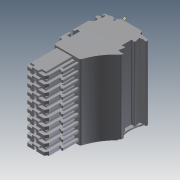
# Autodesk Inventor part: 2010-1201
Saved by Autodesk Inventor 2016 (Build 200138000, 138)
## iProperties
Created: 2014-05-05
Part Number: 2010-1201
Catalog Web Link: www.cadenas.de
Description: 2020-102 TO 2020-115-1-CONDUCTOR FEMALE PLUG for insertion into carrier terminal blocks WITH CODIG FINGERS
Vendor: WAGO
Document SubType Name: Modeling
Designer: PARTuser1
Manufacturer: WAGO
Mass: 22.67 g
Density: 1 g/cm^3
Material: Generic
Appearance: RGB(170.85000425577149,170.85000425577149,170.85000425577149)
Stock Number: 2010-1201
Surface Area: 93.5557 cm^2
Volume: 18.6614 cm^3
Category: PARTsolutions
Company: WAGO
GlobalPropertyList: <PropertyList/>
PSOL_IDENT_0: {$CADENAS_DATA\23d-libs\wago\pg18\serie2020\2020-0102_0999-0962.prj},173 {VTYP=3D},{NB=2020-110},{LI
PSOL_IDENT_1: NA=2020-110},{NN=2020-102 TO 2020-115},{DATE=11.11.2013 10:30:50},{GEOMDATE=15.10.2013 15:25:14},{VE
PSOL_IDENT_2: RSION=},{LINEID=260},{LINESUBID=-1},{WBVAR=}  {NB=2020-110},{LINA=2020-110},{KT=DUMMY},{BESTNR=2020-
PSOL_IDENT_3: 110},{QUERSCHNITT1=0.14 - 1.5},{QUERSCHNITT2=24 - 16},{ABISOLIERLAENGE=9 - 11},{SPANNUNG=500},{BEMES
PSOL_IDENT_4: SSTOSSSPG=6},{VERSCHMUTZGRAD=3},{STROM=13.5},{RM=3.50},{P=10},{HOEHE=40.50},{BREITE=35.00},{TIEFE=20
PSOL_IDENT_5: .70},{ANZAHLKLEMMSTEL=10},{ANZAHLPOTENTIAL=10},{FARBE=grau},{BEMERKUNGEN=L =(No. of poles x Pin Spac
PSOL_IDENT_6: ing},{RGB=0.67,0.67,0.67,0},{GEWICHT=22.670}
CNS_NN: 2020-102 TO 2020-115
CNS_NT: 1-CONDUCTOR FEMALE PLUG for insertion into carrier terminal blocks WITH CODIG FINGERS
CNS_NB: 2020-110
CNS_NBSYN: $BESTNR.
CNS_LINA: 2020-110
CNS_BESTNR: 2020-110
CNS_QUERSCHNITT1: 0.14 - 1.5
CNS_QUERSCHNITT2: 24 - 16
CNS_ABISOLIERLAENGE: 9 - 11
CNS_SPANNUNG: 500
CNS_BEMESSSTOSSSPG: 6
CNS_VERSCHMUTZGRAD: 3
CNS_STROM: 13.5
CNS_RM: 3.50
CNS_P: 10
CNS_HOEHE: 40.50
CNS_BREITE: 35.00
CNS_TIEFE: 20.70
CNS_ANZAHLKLEMMSTEL: 10
CNS_ANZAHLPOTENTIAL: 10
CNS_FARBE: grau
CNS_BEMERKUNGEN: L =(No. of poles x Pin Spacing
CNS_RGB: 0.67,0.67,0.67,0
CNS_GEWICHT: 22.670
SUPPLIER: WAGO
ARTICLENO: 2020-110
BOMINFO: 2020-110
CREATOR: CADENAS GmbH
Title: 2010-1201
Author: Cadenas PARTsolutions
Comments: 1-CONDUCTOR FEMALE PLUG for insertion into carrier terminal blocks WITH CODIG FINGERS
Autodesk Inventor part; units mm, degrees
ref_plane "YZ Plane" through (0, 0, 0) normal (1, 0, 0) x (0, 1, 0)
ref_plane "XZ Plane" through (0, 0, 0) normal (0, 1, 0) x (-1, 0, 0)
ref_plane "XY Plane" through (0, 0, 0) normal (0, 0, 1) x (1, 0, 0)
sketch "Skizze_1" plane through (0, 0, 0) normal (0, 0, 1) x (1, 0, 0)
  arc A0 (-6.5, 18.4245) -> (-5.75, 17.9915) centre (-6, 18.4245) ccw
  line L0 (-5.75, 17.9915) -> (-5.4583, 18.1599)
  arc A1 (-5.1591, 18.0041) -> (-5.4583, 18.1599) centre (-5.3583, 17.9867) ccw
  line L1 (-5.1591, 18.0041) -> (-4.8399, 14.3564)
  arc A2 (-4.8399, 14.3564) -> (-4.3418, 13.9) centre (-4.3418, 14.4) ccw
  line L2 (-4.3418, 13.9) -> (6.9, 13.9)
  arc A3 (6.9, 13.9) -> (7.847, 14.5787) centre (6.9, 14.9) ccw
  arc A4 (15.1547, 25.4441) -> (7.847, 14.5787) centre (31.5214, 6.5462) ccw
  arc A5 (15.1547, 25.4441) -> (15.5, 26.2) centre (14.5, 26.2) ccw
  line L3 (15.5, 26.2) -> (15.5, 26.6)
  arc A6 (15.5, 26.6) -> (14.925, 26.72) centre (15.2, 26.6) ccw
  arc A7 (14.7417, 26.6) -> (14.925, 26.72) centre (14.7417, 26.8) ccw
  line L4 (14.7417, 26.6) -> (14.5, 26.6)
  arc A8 (14.4653, 26.603) -> (14.5, 26.6) centre (14.5, 26.8) ccw
  line L5 (14.4653, 26.603) -> (12.9861, 26.8639)
  arc A9 (12.8277, 27.1126) -> (12.9861, 26.8639) centre (13.0208, 27.0608) ccw
  line L6 (12.8277, 27.1126) -> (13.32, 28.95)
  line L7 (13.32, 28.95) -> (13.32, 29.44)
  arc A10 (13.32, 29.44) -> (12.7085, 29.7795) centre (12.92, 29.44) ccw
  line L8 (12.7085, 29.7795) -> (12.4591, 29.6241)
  arc A11 (11.8535, 29.6935) -> (12.4591, 29.6241) centre (12.2, 30.04) ccw
  line L9 (11.8535, 29.6935) -> (11.7, 29.847)
  line L10 (11.7, 29.847) -> (11.7, 34.053)
  line L11 (11.7, 34.053) -> (11.8535, 34.2065)
  arc A12 (12.4591, 34.2759) -> (11.8535, 34.2065) centre (12.2, 33.86) ccw
  line L12 (12.4591, 34.2759) -> (12.7085, 34.1205)
  arc A13 (12.7085, 34.1205) -> (13.32, 34.46) centre (12.92, 34.46) ccw
  line L13 (13.32, 34.46) -> (13.32, 34.95)
  line L14 (13.32, 34.95) -> (12.8277, 36.7874)
  arc A14 (12.9861, 37.0361) -> (12.8277, 36.7874) centre (13.0208, 36.8392) ccw
  line L15 (12.9861, 37.0361) -> (14.4653, 37.297)
  arc A15 (14.5, 37.3) -> (14.4653, 37.297) centre (14.5, 37.1) ccw
  line L16 (14.5, 37.3) -> (14.8, 37.3)
  arc A16 (14.9765, 37.1941) -> (14.8, 37.3) centre (14.8, 37.1) ccw
  line L17 (14.9765, 37.1941) -> (15.0235, 37.1059)
  arc A17 (15.0235, 37.1059) -> (15.2416, 37.0044) centre (15.2, 37.2) ccw
  line L18 (15.2416, 37.0044) -> (15.6624, 37.0938)
  arc A18 (15.6624, 37.0938) -> (15.9, 37.3873) centre (15.6, 37.3873) ccw
  line L19 (15.9, 37.3873) -> (15.9, 37.5152)
  arc A19 (15.9, 37.5152) -> (14.9872, 38.5114) centre (14.9, 37.5152) ccw
  line L20 (14.9872, 38.5114) -> (11.8147, 38.789)
  arc A20 (10.9359, 39.5263) -> (11.8147, 38.789) centre (11.9018, 39.7852) ccw
  line L21 (10.9359, 39.5263) -> (10.7743, 40.1294)
  arc A21 (10.7743, 40.1294) -> (10.2913, 40.5) centre (10.2913, 40) ccw
  line L22 (10.2913, 40.5) -> (1.35, 40.5)
  line L23 (1.35, 40.5) -> (-3.4, 39.2272)
  line L24 (-3.4, 39.2272) -> (-3.8496, 38.85)
  line L25 (-3.8496, 38.85) -> (-5.1, 38.85)
  arc A22 (-5.1, 38.85) -> (-5.6, 38.35) centre (-5.1, 38.35) ccw
  line L26 (-5.6, 38.35) -> (-5.6, 37.65)
  arc A23 (-5.6, 37.65) -> (-5.4, 37.45) centre (-5.4, 37.65) ccw
  line L27 (-5.4, 37.45) -> (-5.2, 37.45)
  arc A24 (-5.2, 37.45) -> (-5, 37.65) centre (-5.2, 37.65) ccw
  line L28 (-5, 37.65) -> (-5, 37.85)
  arc A25 (-4.8, 38.05) -> (-5, 37.85) centre (-4.8, 37.85) ccw
  line L29 (-4.8, 38.05) -> (-4.6, 38.05)
  arc A26 (-4.4, 37.85) -> (-4.6, 38.05) centre (-4.6, 37.85) ccw
  line L30 (-4.4, 37.85) -> (-4.4, 36.35)
  arc A27 (-4.6, 36.15) -> (-4.4, 36.35) centre (-4.6, 36.35) ccw
  line L31 (-4.6, 36.15) -> (-4.8, 36.15)
  arc A28 (-5, 36.35) -> (-4.8, 36.15) centre (-4.8, 36.35) ccw
  line L32 (-5, 36.35) -> (-5, 36.45)
  arc A29 (-5, 36.45) -> (-5.2, 36.65) centre (-5.2, 36.45) ccw
  line L33 (-5.2, 36.65) -> (-5.5067, 36.65)
  arc A30 (-5.5067, 36.65) -> (-5.6599, 36.5786) centre (-5.5067, 36.45) ccw
  line L34 (-5.6599, 36.5786) -> (-5.7678, 36.45)
  line L35 (-5.7678, 36.45) -> (-6.3, 36.45)
  arc A31 (-6.3, 36.45) -> (-6.5, 36.25) centre (-6.3, 36.25) ccw
  line L36 (-6.5, 36.25) -> (-6.5, 35.45)
  arc A32 (-6.5, 35.45) -> (-6, 34.95) centre (-6, 35.45) ccw
  line L37 (-6, 34.95) -> (-5.3, 34.95)
  arc A33 (-4.8, 34.45) -> (-5.3, 34.95) centre (-5.3, 34.45) ccw
  line L38 (-4.8, 34.45) -> (-4.8, 33.4103)
  arc A34 (-5.0132, 33.0007) -> (-4.8, 33.4103) centre (-5.3, 33.4103) ccw
  line L39 (-5.0132, 33.0007) -> (-6.2868, 32.1089)
  arc A35 (-6.2868, 32.1089) -> (-6.5, 31.6994) centre (-6, 31.6994) ccw
  line L40 (-6.5, 31.6994) -> (-6.5, 24.5)
  arc A36 (-6.5, 24.5) -> (-6.3, 24.3) centre (-6.3, 24.5) ccw
  line L41 (-6.3, 24.3) -> (-5.7, 24.3)
  arc A37 (-5.7, 24.3) -> (-5.5, 24.5) centre (-5.7, 24.5) ccw
  line L42 (-5.5, 24.5) -> (-5.5, 25.4)
  arc A38 (-5.3, 25.6) -> (-5.5, 25.4) centre (-5.3, 25.4) ccw
  line L43 (-5.3, 25.6) -> (-4.3, 25.6)
  arc A39 (-4.1, 25.4) -> (-4.3, 25.6) centre (-4.3, 25.4) ccw
  line L44 (-4.1, 25.4) -> (-4.1, 20.9)
  arc A40 (-4.3, 20.7) -> (-4.1, 20.9) centre (-4.3, 20.9) ccw
  line L45 (-4.3, 20.7) -> (-5.3, 20.7)
  arc A41 (-5.5, 20.9) -> (-5.3, 20.7) centre (-5.3, 20.9) ccw
  line L46 (-5.5, 20.9) -> (-5.5, 22.5)
  arc A42 (-5.5, 22.5) -> (-5.7, 22.7) centre (-5.7, 22.5) ccw
  line L47 (-5.7, 22.7) -> (-6.3, 22.7)
  arc A43 (-6.3, 22.7) -> (-6.5, 22.5) centre (-6.3, 22.5) ccw
  line L48 (-6.5, 22.5) -> (-6.5, 18.4245)
  constraints: 98 end point, 88 point on circle, 44 centre point
extrude "Extrusion1" add sketch "Skizze_1" along normal blind 35
sketch "Skizze_2" plane through (0, 0, 1.925) normal (0, 0, 1) x (1, 0, 0)
  line L0 (-4.45, 1.5) -> (-3.8852, 0.2887)
  arc A0 (-3.8852, 0.2887) -> (-3.432, 0) centre (-3.432, 0.5) ccw
  line L1 (-3.432, 0) -> (4.032, 0)
  arc A1 (4.032, 0) -> (4.4852, 0.2887) centre (4.032, 0.5) ccw
  line L2 (4.4852, 0.2887) -> (5.05, 1.5)
  line L3 (5.05, 1.5) -> (5.05, 13.9)
  line L4 (5.05, 13.9) -> (-4.45, 13.9)
  line L5 (-4.45, 13.9) -> (-4.45, 1.5)
  constraints: 12 end point, 4 point on circle, 2 centre point
extrude "Extrusion2" add sketch "Skizze_2" against normal blind 1.425
pattern_linear "Rectangular Pattern1" count 10 spacing 3.5 along (0, 0, 1) of "Extrusion2"
sketch "Skizze_4" plane through (0, 0, 1.925) normal (0, 0, 1) x (1, 0, 0)
  line L0 (-3.85, 1.5) -> (-3.1505, 0)
  line L1 (-3.1505, 0) -> (3.1505, 0)
  line L2 (3.1505, 0) -> (3.85, 1.5)
  line L3 (3.85, 1.5) -> (3.85, 13.9)
  line L4 (3.85, 13.9) -> (-3.85, 13.9)
  line L5 (-3.85, 13.9) -> (-3.85, 1.5)
  constraints: 12 end point
extrude "Extrusion3" add sketch "Skizze_4" along normal blind 0.825
pattern_linear "Rectangular Pattern2" count 10 spacing 3.5 along (0, 0, 1) of "Extrusion3"
sketch "Skizze_6" plane through (0, 0, 1.925) normal (0, 0, 1) x (1, 0, 0)
  line L0 (-3.85, -1) -> (3.85, -1)
  line L1 (3.85, -1) -> (3.85, 1.5)
  line L2 (3.85, 1.5) -> (1.7144, 1.5)
  line L3 (1.7144, 1.5) -> (1.5, 0.7)
  line L4 (1.5, 0.7) -> (1.5, 0)
  line L5 (1.5, 0) -> (-1.5, 0)
  line L6 (-1.5, 0) -> (-1.5, 0.7)
  line L7 (-1.5, 0.7) -> (-1.7144, 1.5)
  line L8 (-1.7144, 1.5) -> (-3.85, 1.5)
  line L9 (-3.85, 1.5) -> (-3.85, -1)
  constraints: 20 end point
extrude "Extrusion4" cut sketch "Skizze_6" along normal blind 0.825
pattern_linear "Rectangular Pattern3" count 10 spacing 3.5 along (0, 0, 1) of "Extrusion4"
sketch "Skizze_8" plane through (0, 0, 0) normal (0, 1, 0) x (-1, 0, 0)
  line L0 (4, 1.925) -> (4, 3.425)
  line L1 (4, 3.425) -> (-4, 3.425)
  line L2 (-4, 3.425) -> (-4, 1.925)
  line L3 (-4, 1.925) -> (-3.85, 1.925)
  line L4 (-3.85, 1.925) -> (-3.85, 2.35)
  arc A0 (-3.45, 2.75) -> (-3.85, 2.35) centre (-3.45, 2.35) ccw
  line L5 (-3.45, 2.75) -> (3.45, 2.75)
  arc A1 (3.85, 2.35) -> (3.45, 2.75) centre (3.45, 2.35) ccw
  line L6 (3.85, 2.35) -> (3.85, 1.925)
  line L7 (3.85, 1.925) -> (4, 1.925)
  constraints: 16 end point, 4 point on circle, 2 centre point
extrude "Extrusion5" cut sketch "Skizze_8" along normal blind 13.9
pattern_linear "Rectangular Pattern4" count 10 spacing 3.5 along (0, 0, 1) of "Extrusion5"
sketch "Skizze_10" plane through (0, 0, 0) normal (0, 1, 0) x (-1, 0, 0)
  line L0 (0.5, 0.475) -> (0.5, 2.225)
  line L1 (0.5, 2.225) -> (-0.5, 2.225)
  line L2 (-0.5, 2.225) -> (-0.5, 0.475)
  line L3 (-0.5, 0.475) -> (0.5, 0.475)
  constraints: 8 end point
extrude "Extrusion6" cut sketch "Skizze_10" along normal blind 2
pattern_linear "Rectangular Pattern5" count 10 spacing 3.5 along (0, 0, 1) of "Extrusion6"
sketch "Skizze_12" plane through (0, 0, 1.925) normal (0, 0, 1) x (1, 0, 0)
  line L0 (5.08, 7.7) -> (5.08, 6.5)
  line L1 (5.08, 6.5) -> (6, 6.5)
  line L2 (6, 6.5) -> (6, 6.45)
  arc A0 (6, 6.45) -> (6.4, 6.05) centre (6.4, 6.45) ccw
  line L3 (6.4, 6.05) -> (6.6, 6.05)
  arc A1 (6.6, 6.05) -> (7, 6.45) centre (6.6, 6.45) ccw
  line L4 (7, 6.45) -> (7, 7.1878)
  arc A2 (7, 7.8122) -> (7, 7.1878) centre (7.95, 7.5) ccw
  line L5 (7, 7.8122) -> (7, 13.35)
  line L6 (7, 13.35) -> (6.85, 13.5)
  line L7 (6.85, 13.5) -> (6.85, 13.9)
  line L8 (6.85, 13.9) -> (6.15, 13.9)
  line L9 (6.15, 13.9) -> (6.15, 13.5)
  line L10 (6.15, 13.5) -> (6, 13.35)
  line L11 (6, 13.35) -> (6, 7.7)
  line L12 (6, 7.7) -> (5.08, 7.7)
  constraints: 26 end point, 6 point on circle, 3 centre point
extrude "Extrusion7" add sketch "Skizze_12" against normal blind 1.1
pattern_linear "Rectangular Pattern6" count 10 spacing 3.5 along (0, 0, 1) of "Extrusion7"
sketch "Sketch8" plane through (1.35, 40.5, 35) normal (-0.258819, 0.9659258, 0) x (0.9659258, 0.258819, 0)
  point P0 (-2.4, 33.25)
hole "Drilling 1" at (-0.9682, 39.8788, 1.75) direction (0.258819, -0.9659258, 0) diameter 3.6 depth 2 countersink diameter 4.8 countersink angle 90
pattern_linear "Rectangular Pattern7" count 10 spacing 3.5 along (0, 0, 1) of "Drilling 1"
sketch "Skizze_18" plane through (0, 0, 1.75) normal (0, 0, 1) x (1, 0, 0)
  line L0 (1.4794, 40.017) -> (1.8676, 38.5681)
  line L1 (1.8676, 38.5681) -> (4.862, 39.3705)
  line L2 (4.862, 39.3705) -> (4.3444, 41.3023)
  line L3 (4.3444, 41.3023) -> (1.6288, 40.5747)
  line L4 (1.6288, 40.5747) -> (1.4794, 40.017)
  constraints: 10 end point
extrude "Extrusion8" cut sketch "Skizze_18" along normal mid plane 2.55
pattern_linear "Rectangular Pattern8" count 10 spacing 3.5 along (0, 0, 1) of "Extrusion8"
sketch "Skizze_20" plane through (8.4, 0, 0) normal (1, 0, 0) x (0, 0, -1)
  line L0 (-2.5, 40.5) -> (-1.6, 34.7)
  line L1 (-1.6, 34.7) -> (-0.5, 34.7)
  line L2 (-0.5, 34.7) -> (-0.5, 40.5)
  line L3 (-0.5, 40.5) -> (-2.5, 40.5)
  constraints: 8 end point
extrude "Extrusion9" cut sketch "Skizze_20" against normal blind 2.8
pattern_linear "Rectangular Pattern9" count 10 spacing 3.5 along (0, 0, 1) of "Extrusion9"
sketch "Skizze_22" plane through (0, 0, 0) normal (0, 0, 1) x (1, 0, 0)
  line L0 (5.6, 40.5) -> (5.6, 34.7)
  line L1 (5.6, 34.7) -> (7.3, 34.7)
  line L2 (7.3, 34.7) -> (5.6, 40.5)
  constraints: 6 end point
extrude "Extrusion10" add sketch "Skizze_22" along normal blind 35
sketch "Skizze_14" plane through (0, 0, 0) normal (0, 0, 1) x (1, 0, 0)
  arc A0 (-6.5, 18.4245) -> (-5.75, 17.9915) centre (-6, 18.4245) ccw
  line L0 (-5.75, 17.9915) -> (-5.4583, 18.1599)
  arc A1 (-5.1591, 18.0041) -> (-5.4583, 18.1599) centre (-5.3583, 17.9867) ccw
  line L1 (-5.1591, 18.0041) -> (-4.8399, 14.3564)
  arc A2 (-4.8399, 14.3564) -> (-4.3418, 13.9) centre (-4.3418, 14.4) ccw
  line L2 (-4.3418, 13.9) -> (6.9, 13.9)
  arc A3 (6.9, 13.9) -> (7.8567, 14.6089) centre (6.9, 14.9) ccw
  arc A4 (14.0544, 24.9673) -> (7.8567, 14.6089) centre (31.7741, 7.3318) ccw
  arc A5 (14.0544, 24.9673) -> (14.2, 25.32) centre (13.7, 25.32) ccw
  line L3 (14.2, 25.32) -> (14.2, 26.95)
  arc A6 (14.2, 36.95) -> (14.2, 26.95) centre (26.2, 31.95) ccw
  line L4 (14.2, 36.95) -> (14.2, 37.664)
  arc A7 (14.2, 37.664) -> (13.2872, 38.6601) centre (13.2, 37.664) ccw
  line L5 (13.2872, 38.6601) -> (11.8147, 38.789)
  arc A8 (10.9359, 39.5263) -> (11.8147, 38.789) centre (11.9018, 39.7852) ccw
  line L6 (10.9359, 39.5263) -> (10.7743, 40.1294)
  arc A9 (10.7743, 40.1294) -> (10.2913, 40.5) centre (10.2913, 40) ccw
  line L7 (10.2913, 40.5) -> (1.35, 40.5)
  line L8 (1.35, 40.5) -> (-3.4, 39.2272)
  line L9 (-3.4, 39.2272) -> (-3.8496, 38.85)
  line L10 (-3.8496, 38.85) -> (-5.1, 38.85)
  arc A10 (-5.1, 38.85) -> (-5.6, 38.35) centre (-5.1, 38.35) ccw
  line L11 (-5.6, 38.35) -> (-5.6, 37.65)
  arc A11 (-5.6, 37.65) -> (-5.4, 37.45) centre (-5.4, 37.65) ccw
  line L12 (-5.4, 37.45) -> (-5.2, 37.45)
  arc A12 (-5.2, 37.45) -> (-5, 37.65) centre (-5.2, 37.65) ccw
  line L13 (-5, 37.65) -> (-5, 37.85)
  arc A13 (-4.8, 38.05) -> (-5, 37.85) centre (-4.8, 37.85) ccw
  line L14 (-4.8, 38.05) -> (-4.6, 38.05)
  arc A14 (-4.4, 37.85) -> (-4.6, 38.05) centre (-4.6, 37.85) ccw
  line L15 (-4.4, 37.85) -> (-4.4, 36.35)
  arc A15 (-4.6, 36.15) -> (-4.4, 36.35) centre (-4.6, 36.35) ccw
  line L16 (-4.6, 36.15) -> (-4.8, 36.15)
  arc A16 (-5, 36.35) -> (-4.8, 36.15) centre (-4.8, 36.35) ccw
  line L17 (-5, 36.35) -> (-5, 36.45)
  arc A17 (-5, 36.45) -> (-5.2, 36.65) centre (-5.2, 36.45) ccw
  line L18 (-5.2, 36.65) -> (-5.5067, 36.65)
  arc A18 (-5.5067, 36.65) -> (-5.6599, 36.5786) centre (-5.5067, 36.45) ccw
  line L19 (-5.6599, 36.5786) -> (-5.7678, 36.45)
  line L20 (-5.7678, 36.45) -> (-6.3, 36.45)
  arc A19 (-6.3, 36.45) -> (-6.5, 36.25) centre (-6.3, 36.25) ccw
  line L21 (-6.5, 36.25) -> (-6.5, 35.45)
  arc A20 (-6.5, 35.45) -> (-6, 34.95) centre (-6, 35.45) ccw
  line L22 (-6, 34.95) -> (-5.3, 34.95)
  arc A21 (-4.8, 34.45) -> (-5.3, 34.95) centre (-5.3, 34.45) ccw
  line L23 (-4.8, 34.45) -> (-4.8, 33.4103)
  arc A22 (-5.0132, 33.0007) -> (-4.8, 33.4103) centre (-5.3, 33.4103) ccw
  line L24 (-5.0132, 33.0007) -> (-6.2868, 32.1089)
  arc A23 (-6.2868, 32.1089) -> (-6.5, 31.6994) centre (-6, 31.6994) ccw
  line L25 (-6.5, 31.6994) -> (-6.5, 18.4245)
  constraints: 52 end point, 48 point on circle, 24 centre point
extrude "Extrusion11" add sketch "Skizze_14" against normal blind 0.7
sketch "Skizze_15" plane through (0, 0, 0) normal (0, 0, 1) x (1, 0, 0)
  line L0 (-4.45, 13.9) -> (-4.45, 1.5)
  line L1 (-4.45, 1.5) -> (5.05, 1.5)
  line L2 (5.05, 1.5) -> (5.05, 13.9)
  line L3 (5.05, 13.9) -> (-4.45, 13.9)
  constraints: 8 end point
extrude "Extrusion12" add sketch "Skizze_15" along normal blind 0.5
sketch "Sketch14" plane through (-0.4506, 37.947, 5.25) normal (-0.258819, 0.9659258, 0) x (0.9659258, 0.258819, 0)
  arc A0 (-0.4213, 5.25) -> (-0.4213, 1.75) centre (0, 3.5) ccw projected
sketch "Sketch15" plane through (-0.4506, 37.947, 5.25) normal (-0.258819, 0.9659258, 0) x (0.9659258, 0.258819, 0)
  arc A0 (-0.4213, 1.75) -> (-0.4213, -1.75) centre (0, 0) ccw projected
sketch "Sketch16" plane through (-0.4506, 37.947, 5.25) normal (-0.258819, 0.9659258, 0) x (0.9659258, 0.258819, 0)
  arc A0 (-0.4213, -1.75) -> (-0.4213, -5.25) centre (0, -3.5) ccw projected
sketch "Sketch17" plane through (-0.4506, 37.947, 5.25) normal (-0.258819, 0.9659258, 0) x (0.9659258, 0.258819, 0)
  arc A0 (-0.4213, -5.25) -> (-0.4213, -8.75) centre (0, -7) ccw projected
sketch "Sketch18" plane through (-0.4506, 37.947, 5.25) normal (-0.258819, 0.9659258, 0) x (0.9659258, 0.258819, 0)
  arc A0 (-0.4213, -8.75) -> (-0.4213, -12.25) centre (0, -10.5) ccw projected
sketch "Sketch19" plane through (-0.4506, 37.947, 5.25) normal (-0.258819, 0.9659258, 0) x (0.9659258, 0.258819, 0)
  arc A0 (-0.4213, -12.25) -> (-0.4213, -15.75) centre (0, -14) ccw projected
sketch "Sketch20" plane through (-0.4506, 37.947, 5.25) normal (-0.258819, 0.9659258, 0) x (0.9659258, 0.258819, 0)
  arc A0 (-0.4213, -15.75) -> (-0.4213, -19.25) centre (0, -17.5) ccw projected
sketch "Sketch21" plane through (-0.4506, 37.947, 5.25) normal (-0.258819, 0.9659258, 0) x (0.9659258, 0.258819, 0)
  arc A0 (-0.4213, -19.25) -> (-0.4213, -22.75) centre (0, -21) ccw projected
sketch "Sketch22" plane through (-0.4506, 37.947, 5.25) normal (-0.258819, 0.9659258, 0) x (0.9659258, 0.258819, 0)
  arc A0 (-0.4213, -22.75) -> (-0.4213, -26.25) centre (0, -24.5) ccw projected
sketch "Sketch23" plane through (-0.4506, 37.947, 5.25) normal (-0.258819, 0.9659258, 0) x (0.9659258, 0.258819, 0)
  arc A0 (-0.4213, -26.25) -> (-0.4213, -29.75) centre (0, -28) ccw projected
pattern_of_nothing "Rectangular Pattern10"
pattern_of_nothing "Rectangular Pattern11"
body "Solid1"
